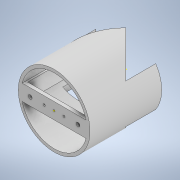
# Autodesk Inventor part: 20220527_仮筒
Saved by Autodesk Inventor 2020 (Build 240168000, 168)
## iProperties
Created: 2022-05-27
Part Number: 20220527_仮筒
Material: 一般
Document SubType Name: Modeling
Designer: Naggy
Density: 1 g/cm^3
Appearance: 既定
Author: Naggy
Autodesk Inventor part; units mm, degrees
ref_plane "YZ Plane" through (0, 0, 0) normal (1, 0, 0) x (0, 1, 0)
ref_plane "XZ Plane" through (0, 0, 0) normal (0, 1, 0) x (-1, 0, 0)
ref_plane "XY Plane" through (0, 0, 0) normal (0, 0, 1) x (1, 0, 0)
sketch "スケッチ1" plane through (0, 0, 0) normal (0, 0, 1) x (1, 0, 0)
  circle A0 centre (0, 0) radius 30
  dimension "d0" = 60
  constraints: 1 centre point, 1 coincident
  measures "d0" diameter of A0
extrude "押し出し1" add sketch "スケッチ1" along normal blind 60
sketch "スケッチ2" plane through (0, 0, 60) normal (0, 0, 1) x (1, 0, 0)
  circle A0 centre (0, 0) radius 26
  dimension "d3" = 52
  constraints: 1 centre point, 1 coincident
  measures "d3" diameter of A0
extrude "押し出し2" cut sketch "スケッチ2" against normal blind 50
sketch "スケッチ3" plane through (0, 0, 0) normal (0, 0, 1) x (1, 0, 0)
  point P0 (0, 0)
sketch "スケッチ4" plane through (0, 0, 0) normal (1, 0, 0) x (0, 1, 0)
  line L0 (30, 0) -> (-30, 0) projected
  line L1 (-30, 0) -> (-30, 60) projected
  arc A0 (30, 0) -> (-30, 0) centre (0, 0) ccw
  dimension "d6" = 30
  constraints: 2 point on circle, 1 centre point, 1 point on line
  measures "d6" radius of A0
extrude "押し出し3" cut sketch "スケッチ4" along normal mid plane 50
sketch "スケッチ5" plane through (0, 0, 60) normal (0, 0, 1) x (1, 0, 0)
  circle A0 centre (0, 0) radius 27.5
  constraints: 1 centre point, 1 coincident
extrude "押し出し4" add sketch "スケッチ5" against normal blind 3
sketch "スケッチ19" plane through (0, 0, 60) normal (0, 0, 1) x (1, 0, 0)
  circle A0 centre (0, 0) radius 27.5
  line L0 (27.5, -6.6575) -> (-27.5, -6.6575)
  line L1 (-27.5, -6.6575) -> (-27.5, 6.6575)
  line L2 (-27.5, 6.6575) -> (27.5, 6.6575)
  line L3 (27.5, 6.6575) -> (27.5, -6.6575)
  line L4 (27.5, -6.6575) -> (-27.5, 6.6575) construction
  line L5 (-27.5, -6.6575) -> (27.5, 6.6575) construction
  point P0 (26.682, -6.6575)
  point P1 (-26.682, -6.6575)
  point P2 (-26.682, 6.6575)
  point P3 (26.682, 6.6575)
  constraints: 12 end point, 2 midpoint, 2 parallel, 1 centre point, 1 coincident, 1 horizontal, 1 perpendicular
extrude "押し出し11" cut sketch "スケッチ19" against normal blind 60 contours L2 A0 | A0 L0
sketch "スケッチ22" plane through (0, 0, 60) normal (0, 0, 1) x (1, 0, 0)
  point P0 (0, 0)
sketch "スケッチ23" plane through (0, 0, 60) normal (0, 0, 1) x (1, 0, 0)
  point P0 (0, 0)
  point P1 (-20, 0)
  point P2 (20, 0)
  dimension "d67" = 20
  dimension "d68" = 20
  measures "d67" distance of point (-20, 0) point (0, 0)
  measures "d68" distance of point (20, 0) point (0, 0)
hole "穴4" at (-20, 0, 60) at (20, 0, 60) direction (0, 0, -1) diameter 3.2 depth 8.8 tip angle 118
sketch "スケッチ25" plane through (0, 0, 60) normal (0, 0, 1) x (1, 0, 0)
  point P0 (0, 0)
  point P1 (0, 0)
  constraints: 1 coincident
hole "穴5" at (0, 0, 60) direction (0, 0, -1) diameter 1.5 depth 8.8 tip angle 118
sketch "スケッチ27" plane through (0, 0, 57) normal (0, 0, -1) x (-1, 0, 0)
  point P0 (0, 0)
  point P1 (8.3, 0)
  point P2 (-8.3, 0)
  dimension "d95" = 8.3
  dimension "d96" = 8.3
  measures "d95" distance of point (8.3, 0) point (0, 0)
  measures "d96" distance of point (0, 0) point (-8.3, 0)
hole "穴7" at (-8.3, 0, 57) at (8.3, 0, 57) direction (0, 0, 1) diameter 1.8 depth 8.8 tip angle 118 counterbore diameter 4 counterbore depth 2
